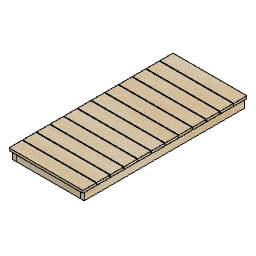
model (Autodesk Fusion 360 design; units mm, degrees)
Autodesk Fusion 360 part; units mm, degrees
sketch "Sketch1" plane through (0, 0, 0) normal (0, 0, 1) x (1, 0, 0) in component "base"
  line L0 (0, 0) -> (762, 0)
  line L1 (762, 0) -> (762, 1708)
  line L2 (762, 1708) -> (0, 1708)
  line L3 (0, 1708) -> (0, 0)
  line L4 (38.1, 38.1) -> (723.9, 38.1)
  line L5 (723.9, 38.1) -> (723.9, 1669.9)
  line L6 (723.9, 1669.9) -> (38.1, 1669.9)
  line L7 (38.1, 1669.9) -> (38.1, 38.1)
  line L8 (38.1, 1669.9) -> (38.1, 1708)
  line L9 (723.9, 1669.9) -> (723.9, 1708)
  line L10 (723.9, 38.1) -> (723.9, 0)
  line L11 (38.1, 38.1) -> (38.1, 0)
  line L12 (400.05, 1669.9) -> (361.95, 1669.9)
  line L13 (361.95, 1669.9) -> (361.95, 38.1)
  line L14 (361.95, 38.1) -> (400.05, 38.1)
  line L15 (400.05, 38.1) -> (400.05, 1669.9)
  line L16 (361.95, 854) -> (38.1, 854) construction
  line L17 (400.05, 854) -> (723.9, 854) construction
  line L18 (400.05, 1335.92) -> (723.9, 1335.92)
  line L19 (723.9, 1335.92) -> (723.9, 1374.02)
  line L20 (723.9, 1374.02) -> (400.05, 1374.02)
  line L21 (400.05, 1374.02) -> (400.05, 1335.92)
  line L22 (38.1, 372.08) -> (361.95, 372.08)
  line L23 (361.95, 372.08) -> (361.95, 333.98)
  line L24 (361.95, 333.98) -> (38.1, 333.98)
  line L25 (38.1, 333.98) -> (38.1, 372.08)
  line L26 (38.1, 1040.04) -> (361.95, 1040.04)
  line L27 (361.95, 1040.04) -> (361.95, 1001.94)
  line L28 (361.95, 1001.94) -> (38.1, 1001.94)
  line L29 (38.1, 1001.94) -> (38.1, 1040.04)
  line L30 (400.05, 706.06) -> (723.9, 706.06)
  line L31 (723.9, 706.06) -> (723.9, 667.96)
  line L32 (723.9, 667.96) -> (400.05, 667.96)
  line L33 (400.05, 667.96) -> (400.05, 706.06)
  line L34 (561.975, 706.06) -> (561.975, 854) construction
  line L35 (200.025, 372.08) -> (561.975, 667.96) construction
  line L36 (561.975, 706.06) -> (200.025, 1001.94) construction
  line L37 (561.975, 667.96) -> (561.975, 38.1) construction
  line L38 (200.025, 333.98) -> (561.975, 38.1) construction
  line L39 (200.025, 1040.04) -> (561.975, 1335.92) construction
  line L40 (200.025, 1040.04) -> (200.025, 1669.9) construction
  line L41 (561.975, 1374.02) -> (200.025, 1669.9) construction
  dimension "d3" = 1708
  dimension "d4" = 762
  dimension "d5" = -38.1
  dimension "d6" = 38.1
  dimension "d7" = 38.1
  dimension "d8" = 38.1
  dimension "d9" = 38.1
  dimension "d10" = 38.1
  constraint horizontal L0
  constraint vertical L1
  constraint horizontal L2
  constraint vertical L3
  constraint coincident L0.start L3.end
  constraint coincident L2 L8.end
  constraint perpendicular L2 L8
  constraint coincident L2 L9.end
  constraint perpendicular L2 L9
  constraint coincident L0 L10.end
  constraint perpendicular L0 L10
  constraint coincident L0 L11.end
  constraint perpendicular L0 L11
  constraint horizontal L12
  constraint vertical L13
  constraint horizontal L14
  constraint vertical L15
  constraint coincident L4 L13.end
  constraint coincident L6 L12.start
  constraint midpoint L13 L16.start
  constraint midpoint L7 L16.end
  constraint midpoint L15 L17.start
  constraint midpoint L5 L17.end
  constraint equal L16 L17
  constraint horizontal L18
  constraint vertical L19
  constraint horizontal L20
  constraint vertical L21
  constraint coincident L5 L19.end
  constraint coincident L15 L18.start
  constraint horizontal L22
  constraint vertical L23
  constraint horizontal L24
  constraint vertical L25
  constraint coincident L13 L23.end
  constraint coincident L7 L22.start
  constraint midpoint L24 L38.start
  constraint horizontal L26
  constraint vertical L27
  constraint horizontal L28
  constraint vertical L29
  constraint coincident L13 L27.end
  constraint coincident L7 L26.start
  constraint horizontal L30
  constraint vertical L31
  constraint horizontal L32
  constraint vertical L33
  constraint coincident L5 L31.end
  constraint coincident L15 L30.start
  constraint midpoint L28 L36.end
  constraint midpoint L30 L34.start
  constraint midpoint L17 L34.end
  constraint perpendicular L17 L34
  constraint midpoint L22 L35.start
  constraint midpoint L32 L35.end
  constraint equal L35 L36
  constraint coincident L4 L37.end
  constraint perpendicular L4 L37
  constraint equal L35 L38
  constraint midpoint L26 L39.start
  constraint midpoint L18 L39.end
  constraint coincident L6 L40.end
  constraint perpendicular L6 L40
  constraint equal L36 L39
  constraint midpoint L20 L41.start
  constraint equal L39 L41
  measures "d3" distance of L0.start L2.end
  measures "d4" distance of L0.start L0.end
  measures "d6" distance of L13.end L14.end
  measures "d7" distance of L22.start L24.end
  measures "d8" distance of L18.end L19.end
  measures "d9" distance of L30.end L31.end
  measures "d10" distance of L26.start L28.end
extrude "Extrude1" add sketch "Sketch1" along normal blind 88.9 contours L0 L4 L10 L11 L14 | L2 L6 L8 L9 L12 | L7 L13 L22 L23 L24 L25 | L5 L15 L30 L31 L32 L33 | L7 L13 L26 L27 L28 L29 | L5 L15 L18 L19 L20 L21 makes body 1 at (146.05, 1040.04, 29.6333) makes body 2 at (266.7, 38.1, 29.6333) makes body 3 at (508, 1335.92, 29.6333) makes body 4 at (615.95, 667.96, 29.6333) makes body 5 at (146.05, 372.08, 29.6333) makes body 6 at (495.3, 1708, 29.6333) in component "base"
extrude "Extrude2" add sketch "Sketch1" along normal blind 88.9 separate body contours L0 L2 L3 L7 L8 L11 L25 L29 | L0 L1 L2 L5 L9 L10 L19 L31 | L4 L6 L12 L13 L14 L15 L21 L23 L27 L33 makes body 7 at (361.95, 1125.9667, 29.6333) makes body 8 at (723.9, 1138.6667, 29.6333) makes body 9 at (0, 1138.6667, 29.6333) in component "base"
sketch "Sketch1 (2)" plane through (0, 0, 88.9) normal (0, 0, 1) x (-1, 0, 0) in component "decking"
  line L0 (-38.1, 0) -> (-38.1, -1708)
  line L1 (-38.1, -1708) -> (0, -1708)
  line L2 (0, -1708) -> (0, 0)
  line L3 (0, 0) -> (-38.1, 0)
  line L4 (12.7, -1720.7) -> (-774.7, -1720.7)
  line L5 (-774.7, -1720.7) -> (-774.7, -1581)
  line L6 (-774.7, -1581) -> (12.7, -1581)
  line L7 (12.7, -1581) -> (12.7, -1720.7)
  line L8 (12.7, -1574.65) -> (-774.7, -1574.65)
  line L9 (-774.7, -1574.65) -> (-774.7, -1434.95)
  line L10 (-774.7, -1434.95) -> (12.7, -1434.95)
  line L11 (12.7, -1434.95) -> (12.7, -1574.65)
  line L12 (12.7, -1428.6) -> (-774.7, -1428.6)
  line L13 (-774.7, -1428.6) -> (-774.7, -1288.9)
  line L14 (-774.7, -1288.9) -> (12.7, -1288.9)
  line L15 (12.7, -1288.9) -> (12.7, -1428.6)
  line L16 (12.7, -1282.55) -> (-774.7, -1282.55)
  line L17 (-774.7, -1282.55) -> (-774.7, -1142.85)
  line L18 (-774.7, -1142.85) -> (12.7, -1142.85)
  line L19 (12.7, -1142.85) -> (12.7, -1282.55)
  line L20 (12.7, -1136.5) -> (-774.7, -1136.5)
  line L21 (-774.7, -1136.5) -> (-774.7, -996.8)
  line L22 (-774.7, -996.8) -> (12.7, -996.8)
  line L23 (12.7, -996.8) -> (12.7, -1136.5)
  line L24 (12.7, -990.45) -> (-774.7, -990.45)
  line L25 (-774.7, -990.45) -> (-774.7, -850.75)
  line L26 (-774.7, -850.75) -> (12.7, -850.75)
  line L27 (12.7, -850.75) -> (12.7, -990.45)
  line L28 (12.7, -844.4) -> (-774.7, -844.4)
  line L29 (-774.7, -844.4) -> (-774.7, -704.7)
  line L30 (-774.7, -704.7) -> (12.7, -704.7)
  line L31 (12.7, -704.7) -> (12.7, -844.4)
  line L32 (12.7, -698.35) -> (-774.7, -698.35)
  line L33 (-774.7, -698.35) -> (-774.7, -558.65)
  line L34 (-774.7, -558.65) -> (12.7, -558.65)
  line L35 (12.7, -558.65) -> (12.7, -698.35)
  line L36 (12.7, -552.3) -> (-774.7, -552.3)
  line L37 (-774.7, -552.3) -> (-774.7, -412.6)
  line L38 (-774.7, -412.6) -> (12.7, -412.6)
  line L39 (12.7, -412.6) -> (12.7, -552.3)
  line L40 (12.7, -406.25) -> (-774.7, -406.25)
  line L41 (-774.7, -406.25) -> (-774.7, -266.55)
  line L42 (-774.7, -266.55) -> (12.7, -266.55)
  line L43 (12.7, -266.55) -> (12.7, -406.25)
  line L44 (12.7, -260.2) -> (-774.7, -260.2)
  line L45 (-774.7, -260.2) -> (-774.7, -120.5)
  line L46 (-774.7, -120.5) -> (12.7, -120.5)
  line L47 (12.7, -120.5) -> (12.7, -260.2)
  line L48 (12.7, -114.15) -> (-774.7, -114.15)
  line L49 (-774.7, -114.15) -> (-774.7, 25.55)
  line L50 (-774.7, 25.55) -> (12.7, 25.55)
  line L51 (12.7, 25.55) -> (12.7, -114.15)
  line L52 (0, -1708) -> (12.7, -1708) construction
  line L53 (-774.7, -1708) -> (-762, -1708) construction
  line L54 (-723.9, -1708) -> (-38.1, -1708) construction
  line L55 (-381, -1708) -> (-381, -1720.7) construction
  point P0 (-762, -1708)
  dimension "d15" = 787.4
  dimension "d16" = 139.7
  dimension "d19" = 0
  dimension "d20" = 146.05
  constraint horizontal L4
  constraint vertical L5
  constraint horizontal L6
  constraint vertical L7
  constraint coincident L1.end L2.start
  constraint coincident L7 L52.end
  constraint perpendicular L7 L52
  constraint coincident L5 L53.start
  constraint coincident P0 L53.end
  constraint perpendicular L5 L53
  constraint equal L52 L53
  constraint midpoint L54 L55.start
  constraint midpoint L4 L55.end
  constraint equal L52 L55
  measures "d15" distance of L4.start L4.end
  measures "d16" distance of L4.end L5.end
extrude "Extrude1'" add sketch "Sketch1 (2)" along normal blind 25.4 separate body contours L0 L2 L3 L48 | L0 L2 L3 L48 L49 L50 L51 | L0 L2 L44 L46 | L0 L44 L45 L46 | L2 L44 L46 L47 | L0 L2 L40 L42 | L0 L40 L41 L42 | L2 L40 L42 L43 | L0 L2 L36 L38 | L0 L36 L37 L38 | L2 L36 L38 L39 | L0 L2 L32 L34 | L0 L32 L33 L34 | L2 L32 L34 L35 | L0 L2 L28 L30 | L0 L28 L29 L30 | L2 L28 L30 L31 | L0 L2 L24 L26 | L0 L24 L25 L26 | L2 L24 L26 L27 | L0 L2 L20 L22 | L0 L20 L21 L22 | L2 L20 L22 L23 | L0 L2 L16 L18 | L0 L16 L17 L18 | L2 L16 L18 L19 | L0 L2 L12 L14 | L0 L12 L13 L14 | L2 L12 L14 L15 | L0 L2 L8 L10 | L0 L8 L9 L10 | L2 L8 L10 L11 | L0 L1 L2 L6 | L0 L1 L2 L4 L5 L6 L7 makes body 10 at (512.2333, 1335.4667, 88.9) makes body 11 at (249.7667, 797.8333, 88.9) makes body 12 at (512.2333, 213.6333, 88.9) makes body 13 at (249.7667, 67.5833, 88.9) makes body 14 at (249.7667, 651.7833, 88.9) makes body 15 at (249.7667, 1235.9833, 88.9) makes body 16 at (512.2333, 1481.5167, 88.9) makes body 17 at (249.7667, 943.8833, 88.9) makes body 18 at (249.7667, 359.6833, 88.9) makes body 19 at (512.2333, 459.1667, 88.9) makes body 20 at (512.2333, 1043.3667, 88.9) makes body 21 at (249.7667, 1674.1333, 88.9) in component "decking"
component "base" placed x (1, 0, 0) y (0, 1, 0) z (0, 0, 1) at (0, 0, 0)
component "decking" placed x (1, 0, 0) y (0, 1, 0) z (0, 0, 1) at (0, 0, 0)
equation "width = 2.5 ft"
equation "length = 1708 mm"
equation "d3 = length"
equation "d4 = width"
equation "d6 = -d5"
equation "d7 = d6"
equation "d8 = d7"
equation "d9 = d8"
equation "d10 = d8"
equation "d15 = width + overhang * 2"
equation "d18 = count"
equation "overhang = 0.5 in"
equation "gap = 0.25 in"
equation "deckingCount = ceil(( length + 2 * overhang ) / 5.75 in)"
equation "count = ceil(deckingCount)"
